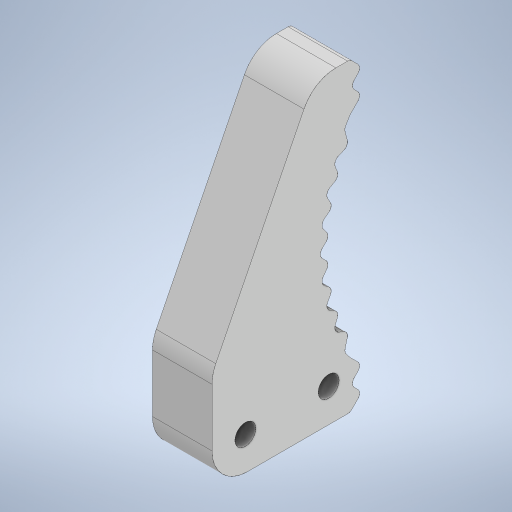
# Autodesk Inventor part: GripperClaw
Saved by Autodesk Inventor 2023 (Build 270158000, 158)
## iProperties
Created: 2023-06-03
Part Number: GripperClaw
Material: Generic
Document SubType Name: Modeling
Designer: komputer
Density: 1 g/cm^3
Appearance: Default
Author: komputer
Autodesk Inventor part; units mm, degrees
ref_plane "YZ Plane" through (0, 0, 0) normal (1, 0, 0) x (0, 1, 0)
ref_plane "XZ Plane" through (0, 0, 0) normal (0, 1, 0) x (-1, 0, 0)
ref_plane "XY Plane" through (0, 0, 0) normal (0, 0, 1) x (1, 0, 0)
sketch "Sketch1" plane through (0, 0, 0) normal (1, 0, 0) x (0, 1, 0)
  line L0 (-0.4351, 18.724) -> (-0.4351, -0.7378)
  arc A0 (40.6729, -0.876) -> (9.4185, -0.876) centre (25.0457, -26.3583) ccw
  line L1 (49.5732, 7.8758) -> (17.5062, 23.9101)
  line L2 (15.3569, 24.324) -> (5.1649, 24.324)
  circle A1 centre (45.9448, 4.2883) radius 1.808
  circle A2 centre (36.1506, 9.2854) radius 1.8018
  circle A3 centre (26.3531, 14.2609) radius 1.7769
  circle A4 centre (16.5584, 19.2972) radius 1.8149
  circle A5 centre (5.1645, 4.724) radius 1.7004
  circle A6 centre (5.1608, 18.7234) radius 1.7042
  line L3 (-0.4351, -0.876) -> (9.4185, -0.876)
  line L4 (40.6729, -0.876) -> (50.8969, -0.876)
  line L5 (50.8969, -0.1885) -> (50.8969, -0.876)
  line L6 (-0.4351, -0.7378) -> (-0.4351, -0.876)
  line L7 (5.529, 24.324) -> (-0.4351, 24.324)
  line L8 (-0.4351, 24.324) -> (-0.4351, 18.724)
  line L9 (15.3569, 24.324) -> (16.6785, 24.324)
  line L10 (17.5062, 23.9101) -> (16.6785, 24.324)
  line L11 (50.8969, -0.876) -> (41.3859, -0.876)
  line L12 (50.8969, 7.2139) -> (50.8969, -0.876)
  line L13 (49.5732, 7.8758) -> (50.8969, 7.2139)
  point P0 (0, 0)
  constraints: 28 end point, 7 centre point, 5 horizontal, 4 collinear, 3 vertical, 2 point on circle, 2 point on line, 1 parallel, 1 perpendicular, 8 other
extrude "Extrusion1" add sketch "Sketch1" along normal blind 10
sketch "Sketch2" plane through (10, 0, 0) normal (1, 0, 0) x (0, 0, -1)
  line L0 (-7.2139, 50.8969) -> (-24.324, 16.6785) projected
  line L1 (-24.324, 16.6785) -> (-24.324, -0.4351) projected
  line L2 (-24.324, -0.4351) -> (0.876, -0.4351) projected
  line L3 (0.876, -0.4351) -> (0.876, 9.4185) projected
  arc A0 (0.876, 40.6729) -> (0.876, 9.4185) centre (26.3583, 25.0457) ccw projected
  line L4 (0.876, 40.6729) -> (0.876, 50.8969) projected
  line L5 (0.876, 50.8969) -> (-7.2139, 50.8969) projected
  circle A1 centre (-4.724, 5.1645) radius 1.7004 projected
  circle A2 centre (-18.7234, 5.1608) radius 1.7042 projected
  circle A3 centre (-4.2883, 45.9448) radius 1.808 projected
  circle A4 centre (-9.2854, 36.1506) radius 1.8018 projected
  circle A5 centre (-19.2972, 16.5584) radius 1.8149 projected
  circle A6 centre (-14.2609, 26.3531) radius 1.7769 projected
  line L6 (-24.324, -0.4351) -> (0.876, -0.4351) projected
  line L7 (0.876, 50.8969) -> (-1.124, 50.8969)
  line L8 (-1.124, 50.8969) -> (-1.124, -0.4351)
  line L9 (-1.124, -0.4351) -> (0.876, -0.4351)
  line L10 (0.876, -0.4351) -> (0.876, 50.8969)
  line L11 (-1.124, 50.8969) -> (1.5326, 50.8969) construction
  line L12 (0.876, 40.6729) -> (0.876, 50.8969) projected
  line L13 (0.876, 48.8969) -> (3.3199, 48.8969) construction
  line L14 (-1.124, 50.8969) -> (0.876, 48.8969)
  line L15 (0.876, 48.8969) -> (-1.124, 46.8969)
  line L16 (-1.124, 46.8969) -> (0.876, 44.8969)
  line L17 (0.876, 44.8969) -> (-1.124, 42.8969)
  line L18 (-1.124, 42.8969) -> (0.876, 40.8969)
  line L19 (0.876, 40.8969) -> (-1.124, 38.8969)
  line L20 (-1.124, 38.8969) -> (0.876, 36.8969)
  line L21 (0.876, 36.8969) -> (-1.124, 34.8969)
  line L22 (-1.124, 34.8969) -> (0.876, 32.8969)
  line L23 (0.876, 32.8969) -> (-1.124, 30.8969)
  line L24 (-1.124, -0.4351) -> (0.876, 1.5649)
  line L25 (-1.124, -0.4351) -> (1.7045, -0.4351) construction
  line L26 (0.876, 1.5649) -> (-1.124, 3.5649)
  line L27 (0.876, 1.5649) -> (3.7045, 1.5649) construction
  line L28 (0.876, 5.5649) -> (-1.124, 7.5649)
  line L29 (-1.124, 3.5649) -> (0.876, 5.5649)
  line L30 (0.876, 9.5649) -> (-1.124, 11.5649)
  line L31 (-1.124, 7.5649) -> (0.876, 9.5649)
  line L32 (0.876, 13.5649) -> (-1.124, 15.5649)
  line L33 (-1.124, 11.5649) -> (0.876, 13.5649)
  line L34 (0.876, 17.5649) -> (-1.124, 19.5649)
  line L35 (-1.124, 15.5649) -> (0.876, 17.5649)
  arc A7 (0.876, 40.6729) -> (0.876, 9.4185) centre (26.3583, 25.0457) ccw projected
  line L36 (26.3583, 25.0457) -> (25.3653, 25.0457)
  line L37 (-3.5341, 25.0457) -> (-4.5271, 25.0457)
  circle A8 centre (25.3653, 25.0457) radius 29.8923
  point P0 (0, 0)
  point P1 (0.2094, 8.8984)
  point P2 (0.876, 7.9042)
  point P3 (0.876, 42.1872)
  point P4 (0.3551, 41.4178)
  dimension "d2" = 2
  dimension "d5" = 45
  dimension "d8" = 45
  dimension "d11" = 4
  dimension "d16" = 45
  dimension "d17" = 135
  dimension "d20" = 4
  dimension "d25" = 0.993
  dimension "d26" = 0.993
  constraints: 60 end point, 7 horizontal, 5 point on line, 2 equal length, 2 parallel, 2 vertical, 1 coincident, 1 perpendicular, 1 point on circle, 43 other
  measures "d2" distance of L9.end L8.end
  measures "d5" angle of L8 L14
  measures "d8" angle of L8 L15
  measures "d11" distance of L7.end L16.start
  measures "d16" angle of L25 L24
  measures "d17" angle of L27 L26
  measures "d20" distance of L24.end L28.start
  measures "d25" distance of L36.start L36.end
  measures "d26" distance of L37.start L37.end
extrude "Extrusion2" cut sketch "Sketch2" against normal blind 10 contours L5 L4 L14 | L15 L4 L16 | L24 L3 L2 | L17 L4 A8 L18 | L29 L3 L26 | L20 A0 L8 | A8 L18 L19 | L19 L4 A0 L20 | L8 A0 L37 A8 | A8 L4 L18 | A8 L3 L10 L4 | L31 A8 L3 L28 | L8 A0 | A0 L20 L21 L8 | A0 L10 L20 | L37 A0 L8 A8 | L8 L30 A0 L31 A8 | L31 A0 L3 A8 | L22 L23 L8 | L21 L10 L22 | L33 A0 L30 | L8 A0 L33 | L31 L10 A0 | A0 L30 L31 | L8 L32 L33 A0 | L23 L10 L34 L8 | A0 L33 L10 L30 | L35 L10 L32 | L8 L34 L35
sketch "Sketch3" plane through (0, 0, 0) normal (-1, 0, 0) x (0, 0, 1)
  arc A0 (-0.2094, 8.8984) -> (-0.3551, 41.4178) centre (-25.3653, 25.0457) ccw projected
  arc A1 (-0.2094, 8.8984) -> (-0.3551, 41.4178) centre (-25.3653, 25.0457) ccw projected
  line L0 (4.5271, 25.0457) -> (6.5271, 25.0457)
  line L1 (6.5271, 25.0457) -> (4.4552, 27.1176)
  line L2 (6.5271, 25.0457) -> (4.4552, 22.9738)
  line L3 (6.2425, 29.2966) -> (4.4653, 26.967)
  line L4 (6.2425, 29.2966) -> (3.913, 31.0738)
  line L5 (5.3939, 33.4715) -> (3.943, 30.9259)
  line L6 (5.3939, 33.4715) -> (2.8483, 34.9224)
  line L7 (3.9964, 37.4962) -> (2.8978, 34.7798)
  line L8 (3.9964, 37.4962) -> (1.2801, 38.5948)
  line L9 (2.075, 41.2986) -> (1.3482, 38.4601)
  line L10 (2.075, 41.2986) -> (-0.7636, 42.0254)
  line L11 (-0.3362, 44.811) -> (-0.6781, 41.9009)
  line L12 (-0.3362, 44.811) -> (-3.2462, 45.153)
  line L13 (-3.1939, 47.9707) -> (-3.145, 45.041)
  line L14 (-3.1939, 47.9707) -> (-6.1236, 47.9217)
  line L15 (-6.4474, 50.7213) -> (-6.0083, 47.8243)
  line L16 (-6.4474, 50.7213) -> (-9.3444, 50.2823)
  line L17 (-10.0384, 53.0137) -> (-9.2171, 50.2011)
  line L18 (-10.0384, 53.0137) -> (-12.851, 52.1925)
  line L19 (-13.9029, 54.807) -> (-12.7141, 52.1289)
  line L20 (-13.9029, 54.807) -> (-16.581, 53.6182)
  line L21 (-17.972, 56.0693) -> (-16.4368, 53.5735)
  line L22 (-17.972, 56.0693) -> (-20.4677, 54.5341)
  line L23 (-22.173, 56.7779) -> (-20.3189, 54.509)
  line L24 (-22.173, 56.7779) -> (-24.4418, 54.9238)
  line L25 (-26.4309, 56.9203) -> (-24.291, 54.9188)
  line L26 (-26.4309, 56.9203) -> (-28.4324, 54.7803)
  line L27 (-30.6699, 56.4938) -> (-28.2822, 54.7954)
  line L28 (-30.6699, 56.4938) -> (-32.3683, 54.1062)
  line L29 (-34.8142, 55.5062) -> (-32.2215, 54.1412)
  line L30 (-34.8142, 55.5062) -> (-36.1792, 52.9135)
  line L31 (-38.7898, 53.975) -> (-36.0383, 52.9677)
  line L32 (-38.7898, 53.975) -> (-39.7971, 51.2235)
  line L33 (-42.526, 51.9275) -> (-39.6647, 51.296)
  line L34 (-42.526, 51.9275) -> (-43.1575, 49.0663)
  line L35 (-45.9558, 49.4004) -> (-43.036, 49.1559)
  line L36 (-45.9558, 49.4004) -> (-46.2004, 46.4805)
  line L37 (-49.0183, 46.4386) -> (-46.0919, 46.5855)
  line L38 (-49.0183, 46.4386) -> (-48.8714, 43.5122)
  line L39 (-51.6586, 43.0951) -> (-48.7779, 43.6307)
  line L40 (-51.6586, 43.0951) -> (-51.1231, 40.2144)
  line L41 (-53.8298, 39.4295) -> (-51.0461, 40.3443)
  line L42 (-53.8298, 39.4295) -> (-52.915, 36.6459)
  line L43 (-55.493, 35.5072) -> (-52.8561, 36.7848)
  line L44 (-55.493, 35.5072) -> (-54.2153, 32.8703)
  line L45 (-56.6185, 31.3982) -> (-54.1755, 33.0159)
  line L46 (-56.6185, 31.3982) -> (-55.0008, 28.9552)
  line L47 (-57.1864, 27.1759) -> (-54.9807, 29.1048)
  line L48 (-57.1864, 27.1759) -> (-55.2575, 24.9703)
  line L49 (-57.1864, 22.9156) -> (-55.2575, 25.1212)
  line L50 (-57.1864, 22.9156) -> (-54.9807, 20.9867)
  line L51 (-56.6185, 18.6932) -> (-55.0008, 21.1363)
  line L52 (-56.6185, 18.6932) -> (-54.1755, 17.0755)
  line L53 (-55.493, 14.5842) -> (-54.2153, 17.2211)
  line L54 (-55.493, 14.5842) -> (-52.8561, 13.3066)
  line L55 (-53.8298, 10.662) -> (-52.915, 13.4456)
  line L56 (-53.8298, 10.662) -> (-51.0461, 9.7472)
  line L57 (-51.6586, 6.9964) -> (-51.1231, 9.8771)
  line L58 (-51.6586, 6.9964) -> (-48.7779, 6.4608)
  line L59 (-49.0183, 3.6528) -> (-48.8714, 6.5792)
  line L60 (-49.0183, 3.6528) -> (-46.0919, 3.506)
  line L61 (-45.9558, 0.6911) -> (-46.2004, 3.6109)
  line L62 (-45.9558, 0.6911) -> (-43.036, 0.9356)
  line L63 (-42.526, -1.8361) -> (-43.1575, 1.0251)
  line L64 (-42.526, -1.8361) -> (-39.6647, -1.2045)
  line L65 (-38.7898, -3.8835) -> (-39.7971, -1.132)
  line L66 (-38.7898, -3.8835) -> (-36.0383, -2.8763)
  line L67 (-34.8142, -5.4147) -> (-36.1792, -2.822)
  line L68 (-34.8142, -5.4147) -> (-32.2215, -4.0497)
  line L69 (-30.6699, -6.4024) -> (-32.3683, -4.0147)
  line L70 (-30.6699, -6.4024) -> (-28.2822, -4.7039)
  line L71 (-26.4309, -6.8288) -> (-28.4324, -4.6888)
  line L72 (-26.4309, -6.8288) -> (-24.291, -4.8273)
  line L73 (-22.173, -6.6864) -> (-24.4418, -4.8323)
  line L74 (-22.173, -6.6864) -> (-20.3189, -4.4176)
  line L75 (-17.972, -5.9778) -> (-20.4677, -4.4427)
  line L76 (-17.972, -5.9778) -> (-16.4368, -3.4821)
  line L77 (-13.9029, -4.7156) -> (-16.581, -3.5268)
  line L78 (-13.9029, -4.7156) -> (-12.7141, -2.0375)
  line L79 (-10.0384, -2.9223) -> (-12.851, -2.101)
  line L80 (-10.0384, -2.9223) -> (-9.2171, -0.1096)
  line L81 (-6.4474, -0.6298) -> (-9.3444, -0.1908)
  line L82 (-6.4474, -0.6298) -> (-6.0083, 2.2672)
  line L83 (-3.1939, 2.1208) -> (-6.1236, 2.1697)
  line L84 (-3.1939, 2.1208) -> (-3.145, 5.0504)
  line L85 (-0.3362, 5.2805) -> (-3.2462, 4.9385)
  line L86 (-0.3362, 5.2805) -> (-0.6781, 8.1905)
  line L87 (2.075, 8.7929) -> (-0.7636, 8.0661)
  line L88 (2.075, 8.7929) -> (1.3482, 11.6314)
  line L89 (3.9964, 12.5953) -> (1.2801, 11.4967)
  line L90 (3.9964, 12.5953) -> (2.8978, 15.3116)
  line L91 (5.3939, 16.6199) -> (2.8483, 15.169)
  line L92 (5.3939, 16.6199) -> (3.943, 19.1656)
  line L93 (6.2425, 20.7949) -> (3.913, 19.0176)
  line L94 (6.2425, 20.7949) -> (4.4653, 23.1245)
  line L95 (1.124, 7.5649) -> (-0.876, 5.5649) projected
  line L96 (-0.2094, 8.8984) -> (1.124, 7.5649) projected
  line L97 (2.075, 8.7929) -> (1.124, 7.5649)
  line L98 (-0.876, 44.8969) -> (1.124, 42.8969) projected
  line L99 (1.124, 42.8969) -> (2.075, 41.2986)
  line L100 (-0.876, 5.5649) -> (-1.6533, 4.7877)
  point P0 (0, 0)
  point P1 (-0.8505, 44.8714)
  point P2 (-3.1467, 45.1413)
  point P3 (-6.0234, 47.9234)
  point P4 (-9.2452, 50.2973)
  point P5 (-12.7548, 52.2206)
  point P6 (-16.4894, 53.6589)
  point P7 (-20.3823, 54.5867)
  point P8 (-24.3642, 54.9873)
  point P9 (-28.3639, 54.8535)
  point P10 (-32.3102, 54.1879)
  point P11 (-36.1325, 53.0022)
  point P12 (-39.7626, 51.3176)
  point P13 (-43.1359, 49.1642)
  point P14 (-46.192, 46.5804)
  point P15 (-48.8765, 43.6124)
  point P16 (-51.1414, 40.313)
  point P17 (-52.9463, 36.7411)
  point P18 (-54.2591, 32.9606)
  point P19 (-55.0562, 29.0388)
  point P20 (-55.3235, 25.0457)
  point P21 (-55.0562, 21.0527)
  point P22 (-54.2591, 17.1309)
  point P23 (-52.9463, 13.3503)
  point P24 (-51.1414, 9.7785)
  point P25 (-48.8765, 6.4791)
  point P26 (-46.192, 3.511)
  point P27 (-43.1359, 0.9272)
  point P28 (-39.7626, -1.2262)
  point P29 (-36.1325, -2.9107)
  point P30 (-32.3102, -4.0964)
  point P31 (-28.3639, -4.7621)
  point P32 (-24.3642, -4.8958)
  point P33 (-20.3823, -4.4952)
  point P34 (-16.4894, -3.5675)
  point P35 (-12.7548, -2.1291)
  point P36 (-9.2452, -0.2058)
  point P37 (-6.0234, 2.168)
  point P38 (-3.1467, 4.9502)
  point P39 (-1.2703, 5.1707)
  point P40 (-0.4228, 6.0181)
  point P41 (-0.6664, 8.0909)
  point P42 (0.3402, 8.3487)
  point P43 (1.3731, 11.5343)
  point P44 (2.9354, 15.2187)
  point P45 (3.9927, 19.0785)
  point P46 (4.5261, 23.0447)
  point P47 (4.5261, 27.0467)
  point P48 (3.9927, 31.013)
  point P49 (2.9354, 34.8728)
  point P50 (1.3731, 38.5572)
  dimension "d29" = 2
  dimension "d30" = 45
  dimension "d31" = 45
  dimension "d34" = 360
  constraints: 196 end point, 3 point on circle, 1 collinear, 236 other
  measures "d29" distance of L0.start L0.end
  measures "d30" angle of L0 L2
  measures "d31" angle of L0 L1
extrude "Extrusion3" cut sketch "Sketch3" against normal blind 10 contours L96 L87 L86 L95 L100 L85 L84 L83 L82 L81 L80 L79 L78 L77 L76 L75 L74 L73 L72 L71 L70 L69 L68 L67 L66 L65 L64 L63 L62 L61 L60 L59 L58 L57 L56 L55 L54 L53 L52 L51 L50 L49 L48 L47 L46 L45 L44 L43 L42 L41 L40 L39 L38 L37 L36 L35 L34 L33 L32 L31 L30 L29 L28 L27 L26 L25 L24 L23 L22 L21 L20 L19 L18 L17 L16 L15 L14 L13 L12 L98 L11 L10 L9 L8 A0 | A0 L89 L88 L87 L96 | A0 L88 L89 | L87 L97 L96 | A0 L91 L90 L89 L88 | A0 L90 L91 | A0 L93 L92 L91 L90 | A0 L92 L93 | A0 L2 L94 L93 L92 | A0 L94 L2 | A0 L0 L2 L94 | A0 L3 L1 L0 | A0 L1 L3 | L1 A0 L5 L4 L3 | A0 L4 L5 | L4 A0 L7 L6 L5 | A0 L6 L7 | L6 A0 L9 L8 L7 | A0 L8 L9 | L10 L11 L98 L99
fillet "Fillet1" radius 6 3 edges at (5, 50.8969, 7.2139) (5, 16.6785, 24.324) (5, -0.4351, 24.324)
fillet "Fillet2" radius 1 27 edges at (5, 50.8969, 1.124) (5, 48.8969, -0.876) (5, 46.8969, 1.124) (5, 44.8969, -0.876) (5, 42.8969, 1.124) (5, 41.2986, 2.075) (5, 38.5572, 1.3731) (5, 37.4962, 3.9964) (5, 34.8728, 2.9354) (5, 33.4715, 5.3939) (5, 31.013, 3.9927) (5, 29.2966, 6.2425) (5, 27.0467, 4.5261) (5, 25.0457, 6.5271) (5, 23.0447, 4.5261) (5, 20.7949, 6.2425) (5, 19.0785, 3.9927) (5, 16.6199, 5.3939) (5, 15.2187, 2.9354) (5, 11.5343, 1.3731) (5, 12.5953, 3.9964) (5, 8.7929, 2.075) (5, 7.5649, 1.124) (5, 5.5649, -0.876) (5, 3.5649, 1.124) (5, 1.5649, -0.876) (5, -0.4351, 1.124)
sketch "Sketch4" plane through (0, 0, 0) normal (-1, 0, 0) x (0, 0, 1)
  circle A0 centre (14.2609, 26.3531) radius 1.7769 projected
  circle A1 centre (19.2972, 16.5584) radius 1.8149 projected
  circle A2 centre (9.2854, 36.1506) radius 1.8018 projected
  circle A3 centre (4.2883, 45.9448) radius 1.808 projected
  circle A4 centre (18.7234, 5.1608) radius 1.7042 projected
  circle A5 centre (4.724, 5.1645) radius 1.7004 projected
  arc A6 (0.8311, -0.1422) -> (1.5382, -0.4351) centre (1.5382, 0.5649) ccw projected
  line L0 (18.324, -0.4351) -> (1.5382, -0.4351) projected
  arc A7 (18.324, -0.4351) -> (24.324, 5.5649) centre (18.324, 5.5649) ccw projected
  line L1 (24.324, 15.262) -> (24.324, 5.5649) projected
  arc A8 (24.324, 15.262) -> (23.6905, 17.9454) centre (18.324, 15.262) ccw projected
  line L2 (8.8723, 47.5803) -> (23.6905, 17.9454) projected
  arc A9 (8.8723, 47.5803) -> (3.5058, 50.8969) centre (3.5058, 44.8969) ccw projected
  line L3 (1.5382, 50.8969) -> (3.5058, 50.8969) projected
  arc A10 (1.5382, 50.8969) -> (0.8311, 50.6041) centre (1.5382, 49.8969) ccw projected
  line L4 (0.8311, 50.6041) -> (-0.1689, 49.6041) projected
  arc A11 (-0.1689, 49.6041) -> (-0.1689, 48.1898) centre (0.5382, 48.8969) ccw projected
  line L5 (-0.1689, 48.1898) -> (0.4169, 47.6041) projected
  arc A12 (0.4169, 46.1898) -> (0.4169, 47.6041) centre (-0.2903, 46.8969) ccw projected
  line L6 (0.4169, 46.1898) -> (-0.1689, 45.6041) projected
  arc A13 (-0.1689, 45.6041) -> (-0.1689, 44.1898) centre (0.5382, 44.8969) ccw projected
  line L7 (-0.1689, 44.1898) -> (1.0356, 42.9853) projected
  arc A14 (1.1879, 42.7895) -> (1.0356, 42.9853) centre (0.3285, 42.2782) ccw projected
  line L8 (1.1879, 42.7895) -> (1.8626, 41.6556) projected
  arc A15 (1.9719, 40.8962) -> (1.8626, 41.6556) centre (1.0032, 41.1442) ccw projected
  line L9 (1.9719, 40.8962) -> (1.59, 39.4044) projected
  arc A16 (1.59, 39.4044) -> (2.1838, 38.2293) centre (2.5587, 39.1563) ccw projected
  line L10 (2.1838, 38.2293) -> (3.0694, 37.8711) projected
  arc A17 (3.6215, 36.5691) -> (3.0694, 37.8711) centre (2.6944, 36.9441) ccw projected
  line L11 (3.6215, 36.5691) -> (3.2633, 35.6835) projected
  arc A18 (3.2633, 35.6835) -> (3.6952, 34.4397) centre (4.1903, 35.3085) ccw projected
  line L12 (3.6952, 34.4397) -> (4.5251, 33.9667) projected
  arc A19 (4.8988, 32.6027) -> (4.5251, 33.9667) centre (4.03, 33.0979) ccw projected
  line L13 (4.8988, 32.6027) -> (4.4257, 31.7728) projected
  arc A20 (4.4257, 31.7728) -> (4.688, 30.4826) centre (5.2945, 31.2776) ccw projected
  line L14 (4.688, 30.4826) -> (5.4475, 29.9031) projected
  arc A21 (5.636, 28.5015) -> (5.4475, 29.9031) centre (4.8409, 29.1081) ccw projected
  line L15 (5.636, 28.5015) -> (5.0565, 27.742) projected
  arc A22 (5.0565, 27.742) -> (5.1445, 26.4283) centre (5.8516, 27.1354) ccw projected
  line L16 (5.1445, 26.4283) -> (5.82, 25.7528) projected
  arc A23 (5.82, 24.3386) -> (5.82, 25.7528) centre (5.1129, 25.0457) ccw projected
  line L17 (5.82, 24.3386) -> (5.1445, 23.6631) projected
  arc A24 (5.1445, 23.6631) -> (5.0565, 22.3495) centre (5.8516, 22.956) ccw projected
  line L18 (5.0565, 22.3495) -> (5.636, 21.5899) projected
  arc A25 (5.4475, 20.1883) -> (5.636, 21.5899) centre (4.8409, 20.9834) ccw projected
  line L19 (5.4475, 20.1883) -> (4.688, 19.6089) projected
  arc A26 (4.688, 19.6089) -> (4.4257, 18.3187) centre (5.2945, 18.8139) ccw projected
  line L20 (4.4257, 18.3187) -> (4.8988, 17.4887) projected
  arc A27 (4.5251, 16.1248) -> (4.8988, 17.4887) centre (4.03, 16.9935) ccw projected
  line L21 (4.5251, 16.1248) -> (3.6952, 15.6517) projected
  arc A28 (3.6952, 15.6517) -> (3.2633, 14.408) centre (4.1903, 14.7829) ccw projected
  line L22 (3.2633, 14.408) -> (3.6215, 13.5223) projected
  arc A29 (3.0694, 12.2203) -> (3.6215, 13.5223) centre (2.6944, 13.1474) ccw projected
  line L23 (3.0694, 12.2203) -> (2.1838, 11.8622) projected
  arc A30 (2.1838, 11.8622) -> (1.59, 10.6871) centre (2.5587, 10.9351) ccw projected
  line L24 (1.59, 10.6871) -> (1.9537, 9.2666) projected
  arc A31 (1.7755, 8.4062) -> (1.9537, 9.2666) centre (0.9849, 9.0186) ccw projected
  line L25 (1.7755, 8.4062) -> (1.1627, 7.615) projected
  arc A32 (1.0792, 7.5202) -> (1.1627, 7.615) centre (0.3721, 8.2273) ccw projected
  line L26 (1.0792, 7.5202) -> (-0.1689, 6.2721) projected
  arc A33 (-0.1689, 6.2721) -> (-0.1689, 4.8578) centre (0.5382, 5.5649) ccw projected
  line L27 (-0.1689, 4.8578) -> (0.4169, 4.2721) projected
  arc A34 (0.4169, 2.8578) -> (0.4169, 4.2721) centre (-0.2903, 3.5649) ccw projected
  line L28 (0.4169, 2.8578) -> (-0.1689, 2.2721) projected
  arc A35 (-0.1689, 2.2721) -> (-0.1689, 0.8578) centre (0.5382, 1.5649) ccw projected
  line L29 (-0.1689, 0.8578) -> (0.8311, -0.1422) projected
  point P0 (0, 0)
extrude "Extrusion4" add sketch "Sketch4" against normal blind 10 contours A0 | A1 | A2 | A3
sketch "Szkic5" plane through (10, 0, 0) normal (1, 0, 0) x (0, 0, -1)
  circle A0 centre (-18.7234, 5.1608) radius 1.7042 projected
  circle A1 centre (-4.724, 5.1645) radius 1.7004 projected
  circle A2 centre (-18.7234, 5.1608) radius 1.75
  circle A3 centre (-4.724, 5.1645) radius 1.75
  point P0 (0, 0)
  dimension "d42" = 3.5
  dimension "d43" = 3.5
  constraints: 2 centre point, 2 coincident
  measures "d42" diameter of A2
  measures "d43" diameter of A3
extrude "Wyciągnięcie proste5" cut sketch "Szkic5" against normal through all contours A0 | A1 | A2 | A3
body "Solid1"
